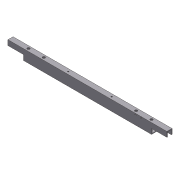
# Autodesk Inventor part: FrameRepresentation_FrontRear
Saved by Autodesk Inventor 2012 (Build 160160000, 160)
## iProperties
Created: 2013-01-06
Part Number: FrameRepresentation_FrontRear
Material: Aluminum-6061
Document SubType Name: Modeling
Designer: JesseK
Mass: 839.613 g
Surface Area: 2005.64 cm^2
Volume: 309.82 cm^3
Density: 2.71 g/cm^3
Author: JesseK
Autodesk Inventor part; units mm, degrees
ref_plane "YZ Plane" through (0, 0, 0) normal (1, 0, 0) x (0, 1, 0)
ref_plane "XZ Plane" through (0, 0, 0) normal (0, 1, 0) x (-1, 0, 0)
ref_plane "XY Plane" through (0, 0, 0) normal (0, 0, 1) x (1, 0, 0)
sketch "Sketch1" plane through (0, 0, 0) normal (0, 0, 1) x (1, 0, 0)
  line L0 (0, 0) -> (787.4, 0)
  line L1 (787.4, 0) -> (787.4, 50.8)
  line L2 (787.4, 50.8) -> (565.5048, 50.8)
  line L3 (565.5048, 50.8) -> (348.1028, 50.8)
  line L4 (348.1028, 50.8) -> (130.7008, 50.8)
  line L5 (130.7008, 50.8) -> (0, 50.8)
  line L6 (0, 50.8) -> (0, 0)
  dimension "d2" = 50.8
  dimension "d3" = 50.8
  dimension "d4" = 787.4
  constraints: 14 end point, 3 horizontal, 2 vertical, 1 collinear
  measures "d2" distance between parallel lines of L0 L5
  measures "d3" distance of L0.end L1.end
  measures "d4" distance of L0.end L0.start
extrude "Extrusion1" add sketch "Sketch1" along normal blind 25.4
shell "Shell1" thickness 3.175 removed faces 2 at (0, 33.8667, 16.9333) at (787.4, 16.9333, 16.9333)
sketch "Sketch2" plane through (0, 0, 25.4) normal (0, 0, 1) x (1, 0, 0)
  line L0 (0, 0) -> (76.2, 0)
  line L1 (76.2, 0) -> (76.2, 25.4)
  line L2 (76.2, 25.4) -> (0, 25.4)
  line L3 (0, 25.4) -> (0, 0)
  line L4 (787.4, 0) -> (711.2, 0)
  line L5 (711.2, 0) -> (711.2, 25.4)
  line L6 (711.2, 25.4) -> (787.4, 25.4)
  line L7 (787.4, 25.4) -> (787.4, 0)
  dimension "d9" = 25.4
  dimension "d12" = 76.2
  constraints: 16 end point, 4 parallel, 2 equal length, 2 horizontal, 2 perpendicular
  measures "d9" distance of L4.end L5.end
  measures "d12" distance of L1.end L2.end
extrude "Extrusion2" cut sketch "Sketch2" against normal through all
sketch "Sketch4" plane through (0, 50.8, 0) normal (0, 1, 0) x (1, 0, 0)
  line L0 (787.4, 0) -> (787.4, -25.4) projected
  line L1 (787.4, 0) -> (0, 0) projected
  circle A0 centre (501.65, -12.7) radius 3.175
  circle A1 centre (285.75, -12.7) radius 3.175
  dimension "d21" = 285.75
  dimension "d22" = 215.9
  dimension "d23" = 12.7
  dimension "d24" = 12.7
  dimension "d25" = 6.35
  dimension "d26" = 6.35
  constraints: 2 centre point
  measures "d21" distance from line of L0 A0.centre
  measures "d22" distance of A0.centre A1.centre
  measures "d23" distance from line of L1 A0.centre
  measures "d24" distance from line of L1 A1.centre
  measures "d25" diameter of A1
  measures "d26" diameter of A0
extrude "Extrusion4" cut sketch "Sketch4" against normal through all
sketch "Sketch5" plane through (76.2, 0, 0) normal (0, -1, 0) x (1, 0, 0)
  circle A0 centre (209.55, 12.7) radius 3.175 projected
  circle A1 centre (425.45, 12.7) radius 3.175 projected
  circle A2 centre (209.55, 12.7) radius 6.35
  circle A3 centre (425.45, 12.7) radius 6.35
  point P0 (-76.2, 0)
  dimension "d29" = 12.7
  dimension "d30" = 12.7
  constraints: 2 centre point, 2 coincident
  measures "d29" diameter of A3
  measures "d30" diameter of A2
extrude "Extrusion5" cut sketch "Sketch5" against normal up to next
sketch "Sketch6" plane through (76.2, 0, 0) normal (0, -1, 0) x (1, 0, 0)
  line L0 (635, 25.4) -> (0, 25.4) projected
  circle A0 centre (12.6948, 12.7) radius 3.175
  circle A1 centre (88.8948, 12.7) radius 3.175
  circle A2 centre (546.1057, 12.7) radius 3.175
  circle A3 centre (622.3057, 12.7) radius 3.175
  line L1 (711.2, 22.225) -> (711.2, 3.175) projected
  line L2 (-76.2, 3.175) -> (-76.2, 22.225) projected
  point P0 (-76.2, 0)
  dimension "d33" = 88.8943
  dimension "d34" = 76.2
  dimension "d35" = 6.35
  dimension "d36" = 12.7
  dimension "d37" = 12.7
  dimension "d38" = 12.7
  dimension "d39" = 12.7
  dimension "d40" = 88.8948
  dimension "d41" = 76.2
  constraints: 4 centre point, 3 equal radius
  measures "d33" distance from line of L1 A3.centre
  measures "d34" distance of A2.centre A3.centre
  measures "d35" diameter of A3
  measures "d36" distance from line of L0 A3.centre
  measures "d37" distance from line of L0 A2.centre
  measures "d38" distance from line of L0 A1.centre
  measures "d39" distance from line of L0 A0.centre
  measures "d40" distance from line of A0.centre L2
  measures "d41" distance of A1.centre A0.centre
extrude "Extrusion6" cut sketch "Sketch6" against normal through all
sketch "Sketch7" plane through (0, 50.8, 0) normal (0, 1, 0) x (1, 0, 0)
  circle A0 centre (698.5057, -12.7) radius 3.175 projected
  circle A1 centre (622.3057, -12.7) radius 3.175 projected
  circle A2 centre (165.0948, -12.7) radius 3.175 projected
  circle A3 centre (88.8948, -12.7) radius 3.175 projected
  circle A4 centre (698.5057, -12.7) radius 6.35
  circle A5 centre (622.3057, -12.7) radius 6.35
  circle A6 centre (88.8948, -12.7) radius 6.35
  circle A7 centre (165.0948, -12.7) radius 6.35
  dimension "d44" = 12.7
  constraints: 4 centre point, 4 coincident, 3 equal radius
  measures "d44" diameter of A6
extrude "Extrusion7" cut sketch "Sketch7" against normal up to next
sketch "Sketch8" plane through (0, 0, 25.4) normal (0, 0, 1) x (1, 0, 0)
  line L0 (787.4, 50.8) -> (787.4, 25.4) projected
  line L1 (0, 50.8) -> (787.4, 50.8) projected
  circle A0 centre (631.825, 34.925) radius 3.175
  circle A1 centre (660.4, 34.925) radius 3.175
  line L2 (631.825, 34.925) -> (660.4, 34.925) construction
  line L3 (0, 25.4) -> (0, 50.8) projected
  line L4 (631.825, 34.925) -> (155.575, 34.925) construction
  line L5 (155.575, 34.925) -> (127, 34.925) construction
  line L6 (127, 34.925) -> (0, 34.925) construction
  circle A2 centre (127, 34.925) radius 3.175
  circle A3 centre (155.575, 34.925) radius 3.175
  point P0 (0, 0)
  dimension "d47" = 127
  dimension "d48" = 28.575
  dimension "d49" = 15.875
  dimension "d50" = 6.35
  dimension "d53" = 127
  dimension "d54" = 28.575
  dimension "d55" = 476.25
  constraints: 8 end point, 4 centre point, 4 horizontal, 3 equal radius, 2 coincident, 1 point on line
  measures "d47" distance from line of L0 L2.end
  measures "d48" distance of L2.end L2.start
  measures "d49" distance from line of L1 L2.end
  measures "d50" diameter of A0
  measures "d53" distance from line of L3 A2.centre
  measures "d54" distance of A3.centre A2.centre
  measures "d55" distance of L2.start L4.end
extrude "Extrusion8" cut sketch "Sketch8" against normal through all
sketch "Sketch9" plane through (0, 0, 25.4) normal (0, 0, 1) x (1, 0, 0)
  circle A0 centre (155.575, 34.925) radius 3.175 projected
  circle A1 centre (127, 34.925) radius 3.175 projected
  circle A2 centre (660.4, 34.925) radius 3.175 projected
  circle A3 centre (631.825, 34.925) radius 3.175 projected
  circle A4 centre (631.825, 34.925) radius 6.35
  circle A5 centre (660.4, 34.925) radius 6.35
  circle A6 centre (127, 34.925) radius 6.35
  circle A7 centre (155.575, 34.925) radius 6.35
  point P0 (0, 0)
  dimension "d56" = 12.7
  constraints: 4 centre point, 4 coincident, 3 equal radius
  measures "d56" diameter of A6
extrude "Extrusion9" cut sketch "Sketch9" against normal up to next
body "Solid1"
